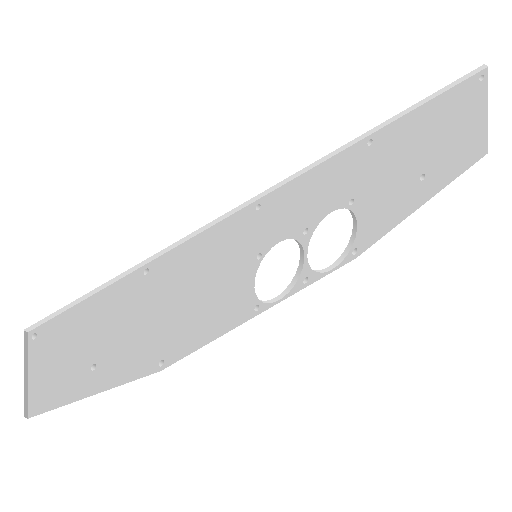
# Autodesk Inventor part: InsideChassiPlate3.0
Saved by Autodesk Inventor 2023 (Build 270158000, 158)
## iProperties
Created: 2022-09-18
Part Number: InsideChassiPlate3.0
Material: Generic
Document SubType Name: Modeling
Designer: deli
Density: 1 g/cm^3
Appearance: Default
Mass: 76.7316 g
Surface Area: 518.075 cm^2
Volume: 76.7316 cm^3
Author: deli
Autodesk Inventor part; units mm, degrees
ref_plane "YZ Plane" through (0, 0, 0) normal (1, 0, 0) x (0, 1, 0)
ref_plane "XZ Plane" through (0, 0, 0) normal (0, 1, 0) x (-1, 0, 0)
ref_plane "XY Plane" through (0, 0, 0) normal (0, 0, 1) x (1, 0, 0)
sketch "Sketch1" plane through (0, 0, 0) normal (1, 0, 0) x (0, 1, 0)
  line L0 (153.267, 41.7419) -> (153.267, -105.149) projected
  arc A0 (153.267, -105.149) -> (153.3544, -106.0799) centre (158.267, -105.149) ccw projected
  line L1 (153.3544, -106.0799) -> (172.4208, -206.7036) projected
  line L2 (172.4208, -206.7036) -> (253.267, -206.7036) projected
  line L3 (253.267, 80.7753) -> (253.267, 143.2964) projected
  line L4 (253.267, 143.2964) -> (172.4208, 143.2964) projected
  line L5 (172.4208, 143.2964) -> (153.3544, 42.6727) projected
  arc A1 (153.3544, 42.6727) -> (153.267, 41.7419) centre (158.267, 41.7419) ccw projected
  circle A2 centre (224.267, 53.2964) radius 2 projected
  circle A3 centre (224.267, -116.7036) radius 2 projected
  circle A4 centre (192.186, -102.5532) radius 2 projected
  circle A5 centre (158.267, -30.806) radius 2 projected
  circle A6 centre (157.883, -67.9775) radius 2 projected
  circle A7 centre (190.1509, -67.9775) radius 2 projected
  circle A8 centre (174.017, -88.0464) radius 7 construction
  circle A9 centre (174.017, -47.9087) radius 7 construction
  circle A10 centre (181.267, -156.7036) radius 2 projected
  circle A11 centre (181.267, 93.2964) radius 2 projected
  circle A12 centre (224.267, 138.2964) radius 2 projected
  circle A13 centre (191.4689, -32.5466) radius 2 projected
  circle A14 centre (224.267, -31.7036) radius 2 projected
  circle A15 centre (158.267, 41.7419) radius 2 projected
  circle A16 centre (158.267, -105.149) radius 2 projected
  circle A17 centre (224.267, -201.7036) radius 2 projected
  circle A18 centre (224.267, -201.7036) radius 2 projected
  line L6 (229.267, 143.2964) -> (229.267, -206.7036)
  line L7 (525.9265, -92.3836) -> (254.1996, 79.0839) projected
  circle A19 centre (508.1, -92.9591) radius 1.5 projected
  circle A20 centre (393.9306, -20.9149) radius 1.5 projected
  circle A21 centre (279.7613, 51.1292) radius 1.5 projected
  circle A22 centre (174.017, -47.9087) radius 19
  circle A23 centre (174.017, -88.0464) radius 19
  line L8 (253.267, -206.7036) -> (580.2998, -118.9663) projected
  arc A24 (580.2998, -118.9663) -> (580.5697, -111.3223) centre (579.2633, -115.1029) ccw projected
  line L9 (580.5697, -111.3223) -> (526.3406, -92.5825) projected
  arc A25 (525.9265, -92.3836) -> (526.3406, -92.5825) centre (526.9939, -90.6922) ccw projected
  arc A26 (253.267, 80.7753) -> (254.1996, 79.0839) centre (255.267, 80.7753) ccw projected
  circle A27 centre (579.2633, -115.1029) radius 1.6 projected
  point P0 (0, 0)
  dimension "d10" = 5
  dimension "d13" = 38
  constraints: 2 centre point, 2 coincident, 2 end point, 2 point on line, 1 equal radius, 1 vertical
  measures "d10" distance from line of L6 A14.centre
  measures "d13" diameter of A22
extrude "Extrusion1" add sketch "Sketch1" along normal blind 3.175 contours A1 L5 L4 L6 L2 L1 A0 L0
body "Solid1"
